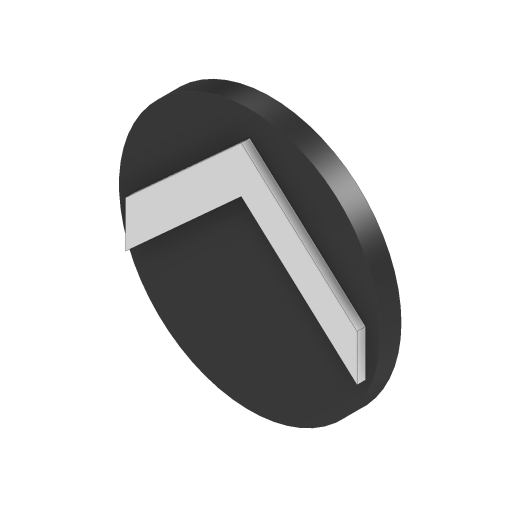
# Autodesk Inventor part: button_plate_arrow
Saved by Autodesk Inventor 2023 (Build 270158000, 158)
## iProperties
Created: 2025-02-19
Part Number: button_plate_arrow
Material: Všeobecné
Document SubType Name: Modeling
Designer: Marek
Density: 1 g/cm^3
Appearance: Výchozí
Author: Marek
Autodesk Inventor part; units mm, degrees
ref_plane "YZ Plane" through (0, 0, 0) normal (1, 0, 0) x (0, 1, 0)
ref_plane "XZ Plane" through (0, 0, 0) normal (0, 1, 0) x (-1, 0, 0)
ref_plane "XY Plane" through (0, 0, 0) normal (0, 0, 1) x (1, 0, 0)
sketch "Náčrt1" plane through (0, 0, 0) normal (0, 0, 1) x (1, 0, 0)
  line L0 (0, 8.68) -> (0, -8.68) projected
  line L1 (-8.68, 0) -> (8.68, 0) projected
  circle A0 centre (0, 0) radius 6.2
  dimension "d0" = 12.4
  constraints: 1 centre point, 1 coincident
  measures "d0" diameter of A0
extrude "Vysunutí1" add sketch "Náčrt1" along normal blind 1
sketch "Náčrt2" plane through (0, 0, 1) normal (0, 0, 1) x (1, 0, 0)
  line L0 (-8.68, 0) -> (8.68, 0) projected
  line L1 (0, 8.68) -> (0, -8.68) projected
  line L2 (-5.5, 0) -> (-5.5, -2.2)
  line L3 (-5.5, -2.2) -> (0, 2.8)
  line L4 (-5.5, 0) -> (0, 5)
  line L5 (5.5, 0) -> (0, 5)
  line L6 (0, 2.8) -> (5.5, -2.2)
  line L7 (5.5, -2.2) -> (5.5, 0)
  point P0 (0, 0)
  dimension "d3" = 2.2
  dimension "d4" = 2.2
  dimension "d5" = 5.5
  dimension "d6" = 5.5
  dimension "d7" = 5
  dimension "d8" = 2.2
  constraints: 12 end point, 4 point on line, 1 perpendicular, 1 vertical
  measures "d3" distance from line of L2.end L0
  measures "d4" distance from line of L6.end L0
  measures "d5" distance between parallel lines of L1 L2
  measures "d6" distance between parallel lines of L1 L7
  measures "d7" distance from line of L0 L4.end
  measures "d8" distance of L4.end L3.end
extrude "Vysunutí2" add sketch "Náčrt2" along normal blind 0.4 contours L4 L1 L3 L0 | L0 L3 L2 | L5 L0 L6 L1 | L7 L6 L0
